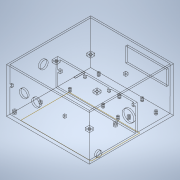
# Autodesk Inventor part: Base
Saved by Autodesk Inventor 2022.2 (Build 262287000, 287)
## iProperties
Created: 2022-01-15
Part Number: Base
Material: Generic
Document SubType Name: Modeling
Designer: siwat
Density: 1 g/cm^3
Appearance: Default
Author: siwat
Autodesk Inventor part; units mm, degrees
ref_plane "YZ Plane" through (0, 0, 0) normal (1, 0, 0) x (0, 1, 0)
ref_plane "XZ Plane" through (0, 0, 0) normal (0, 1, 0) x (-1, 0, 0)
ref_plane "XY Plane" through (0, 0, 0) normal (0, 0, 1) x (1, 0, 0)
ref_plane "Work Plane1" through (31.5112, 10.0003, 59.575) normal (-0.0015858, -0.9999987, 0.0000018) x (-0.0011293, 0, -0.9999994)
sketch "Sketch1" plane through (31.5112, 10.0003, 59.575) normal (-0.0015858, -0.9999987, 0.0000018) x (-0.0011293, 0, -0.9999994)
  line L0 (-4.5224, 4.5326) -> (134.4396, 4.5326)
  line L1 (134.4396, 4.5326) -> (134.4396, -131.8992)
  line L2 (134.4396, -131.8992) -> (-4.5224, -131.8992)
  line L3 (-4.5224, -131.8992) -> (-4.5224, 4.5326)
  line L4 (-7.5224, 7.5326) -> (137.4396, 7.5326)
  line L5 (137.4396, 7.5326) -> (137.4396, -134.8992)
  line L6 (137.4396, -134.8992) -> (-7.5224, -134.8992)
  line L7 (-7.5224, -134.8992) -> (-7.5224, 7.5326)
  point P0 (59.6106, -31.428)
  dimension "d0" = 138.9621
  dimension "d1" = 136.4319
  dimension "d2" = 74.8291
  dimension "d3" = 35.9607
  dimension "d4" = 3
  dimension "d5" = 3
  dimension "d6" = 3
  dimension "d7" = 3
  constraints: 16 end point, 4 parallel, 2 horizontal, 2 perpendicular
  measures "d0" distance between parallel lines of L1 L3
  measures "d1" distance between parallel lines of L0 L2
  measures "d2" distance from line of point (59.611, -31.428) L1
  measures "d3" distance from line of point (59.611, -31.428) L0
  measures "d4" distance between parallel lines of L0 L4
  measures "d5" distance between parallel lines of L3 L7
  measures "d6" distance between parallel lines of L5 L1
  measures "d7" distance between parallel lines of L6 L2
extrude "Extrusion1" add sketch "Sketch1" against normal blind 74.125
sketch "Sketch2" plane through (31.5112, 10.0003, 59.575) normal (-0.0015858, -0.9999987, 0.0000018) x (0.9999981, -0.0015858, -0.0011293)
  line L0 (-134.8992, -137.4396) -> (7.5326, -137.4396) projected
  line L1 (7.5326, 7.5224) -> (-134.8992, 7.5224) projected
  line L2 (7.5326, -137.4396) -> (-134.8992, -137.4396)
  line L3 (-134.8992, -137.4396) -> (-134.8992, 7.5224)
  line L4 (-134.8992, 7.5224) -> (7.5326, 7.5224)
  line L5 (7.5326, 7.5224) -> (7.5326, -137.4396)
  point P0 (-31.428, -59.6106)
  point P1 (-134.8992, -137.4396)
  point P2 (7.5326, 7.5224)
  constraints: 8 end point, 2 parallel, 1 horizontal, 1 perpendicular
extrude "Extrusion2" add sketch "Sketch2" along normal blind 3
sketch "Sketch3" plane through (31.5112, 10.0003, 59.575) normal (0.0015858, 0.9999987, -0.0000018) x (0.9999981, -0.0015858, -0.0011293)
  circle A0 centre (-112.8782, 129.2967) radius 1.9965
  circle A1 centre (-112.8782, 129.2967) radius 0.875
  circle A2 centre (-114.2274, 81.024) radius 1.9965
  circle A3 centre (-114.2274, 81.024) radius 0.875
  circle A4 centre (-62.1401, 86.0453) radius 1.9965
  circle A5 centre (-62.1401, 86.0453) radius 0.875
  circle A6 centre (-62.0938, 113.9832) radius 1.9965
  circle A7 centre (-62.0938, 113.9832) radius 0.875
  circle A8 centre (-37.9957, 129.2347) radius 1.9965
  circle A9 centre (-37.9957, 129.2347) radius 0.875
  circle A10 centre (-31.6312, 80.9446) radius 1.9965
  circle A11 centre (-31.6312, 80.9446) radius 0.875
  circle A12 centre (-6.6551, 121.5212) radius 2.3058
  circle A13 centre (-6.6551, 121.5212) radius 0.875
  circle A14 centre (-22.9352, 91.3493) radius 2.3058
  circle A15 centre (-22.9352, 91.3493) radius 0.875
  circle A16 centre (-129.08, 0.6108) radius 2.6932
  circle A17 centre (-129.08, 0.6108) radius 0.875
  circle A18 centre (-24.0772, 69.1234) radius 2.8442
  circle A19 centre (-24.0772, 69.1234) radius 0.875
  point P0 (-31.428, 59.6106)
  dimension "d12" = 1.75
  dimension "d13" = 1.75
  dimension "d14" = 1.75
  dimension "d15" = 1.75
  dimension "d16" = 1.75
  dimension "d17" = 1.75
  dimension "d18" = 1.75
  dimension "d19" = 1.75
  dimension "d28" = 1.75
  dimension "d29" = 1.75
  constraints: 20 centre point, 10 coincident
  measures "d12" diameter of A1
  measures "d13" diameter of A3
  measures "d14" diameter of A5
  measures "d15" diameter of A7
  measures "d16" diameter of A9
  measures "d17" diameter of A11
  measures "d18" diameter of A13
  measures "d19" diameter of A15
  measures "d28" diameter of A17
  measures "d29" diameter of A19
extrude "Extrusion3" add sketch "Sketch3" along normal blind 5
sketch "Sketch4" plane through (31.5112, 10.0003, 59.575) normal (0.0015858, 0.9999987, -0.0000018) x (0.9999981, -0.0015858, -0.0011293)
  line L0 (4.5326, 134.4396) -> (4.5326, -4.5224) projected
  line L1 (-131.8992, 134.4396) -> (-131.8992, -4.5224) projected
  line L2 (4.5326, 74.8611) -> (-131.8992, 74.8611)
  line L3 (-131.8992, 74.8611) -> (-131.8992, 77.8611)
  line L4 (-131.8992, 77.8611) -> (4.5326, 77.8611)
  line L5 (4.5326, 77.8611) -> (4.5326, 74.8611)
  point P0 (-31.428, 59.6106)
  point P1 (4.5326, 77.8611)
  point P2 (-131.8992, 74.8611)
  dimension "d22" = 3
  constraints: 8 end point, 2 parallel, 2 point on line, 1 horizontal, 1 perpendicular
  measures "d22" distance between parallel lines of L4 L2
extrude "Extrusion4" add sketch "Sketch4" along normal blind 45
sketch "Sketch5" plane through (35.9559, 9.9931, -18.2911) normal (-0.0011293, 0, -0.9999994) x (-0.9999981, 0.0015858, 0.0011293)
  circle A0 centre (12.779, 19.6609) radius 10
  point P0 (35.9607, -10.0501)
  dimension "d25" = 20
  constraints: 1 centre point
  measures "d25" diameter of A0
extrude "Extrusion5" cut sketch "Sketch5" against normal up to surface (3 mm away)
sketch "Sketch7" plane through (-100.5396, 10.2094, -74.7156) normal (0.9999981, -0.0015858, -0.0011293) x (-0.0011293, 0, -0.9999994)
  line L0 (0, 0) -> (0, 74.125) projected
  line L1 (0, 24.9377) -> (-4, 24.9377)
  line L2 (-4, 24.9377) -> (-4, 20.9377)
  line L3 (-4, 20.9377) -> (0, 20.9377)
  line L4 (0, 20.9377) -> (0, 24.9377)
  line L5 (-4, 24.9377) -> (-56.5786, 24.9377)
  line L6 (-56.5786, 45) -> (-56.5786, 0) projected
  line L7 (-4, 20.9377) -> (-56.5786, 20.9377)
  line L8 (-52.5786, 24.9377) -> (-52.5786, 20.9377)
  line L9 (-56.5786, 0) -> (-56.5786, 45) projected
  point P0 (-74.8291, -10.0501)
  point P1 (-56.5786, 90)
  dimension "d30" = 4
  dimension "d31" = 4
  dimension "d34" = 4
  constraints: 15 end point, 4 point on line, 3 horizontal, 2 parallel, 2 perpendicular
  measures "d30" distance of L3.end L2.end
  measures "d31" distance of L2.end L1.end
  measures "d34" distance from line of L6.start L8
extrude "Extrusion6" add sketch "Sketch7" along normal blind 4 contours L3 L2 L1 L0 | L7 L6 L5 L8
sketch "Sketch8" plane through (-100.4955, 35.1471, -70.7156) normal (0.0015858, 0.9999987, -0.0000018) x (0.9999981, -0.0015858, -0.0011293)
  line L0 (136.4319, 4) -> (136.4319, -134.9621) projected
  line L1 (136.4319, 4) -> (129.4319, 4)
  line L2 (129.4319, 4) -> (129.4319, -3)
  line L3 (129.4319, -3) -> (136.4319, -3)
  line L4 (136.4319, -3) -> (136.4319, 4)
  line L5 (136.4319, -52.5786) -> (132.4319, -52.5786)
  line L6 (132.4319, -52.5786) -> (132.4319, -48.5786)
  line L7 (132.4319, -48.5786) -> (136.4319, -48.5786)
  line L8 (136.4319, -48.5786) -> (136.4319, -52.5786)
  line L9 (136.4319, 4) -> (0, 4) projected
  line L10 (60.4128, 4) -> (64.4128, 4)
  line L11 (64.4128, 4) -> (64.4128, 0)
  line L12 (64.4128, 0) -> (60.4128, 0)
  line L13 (60.4128, 0) -> (60.4128, 4)
  line L14 (0, -52.5786) -> (136.4319, -52.5786) projected
  line L15 (60.4128, -52.5786) -> (67.4128, -52.5786)
  line L16 (67.4128, -52.5786) -> (67.4128, -45.5786)
  line L17 (67.4128, -45.5786) -> (60.4128, -45.5786)
  line L18 (60.4128, -45.5786) -> (60.4128, -52.5786)
  circle A0 centre (132.9319, 0.5) radius 1.25
  circle A1 centre (63.9128, -49.0786) radius 1.25
  point P0 (100.4712, -70.8291)
  point P1 (67.4128, -52.5786)
  point P2 (64.4128, 4)
  dimension "d35" = 7
  dimension "d36" = 7
  dimension "d37" = 4
  dimension "d38" = 4
  dimension "d39" = 4
  dimension "d40" = 4
  dimension "d41" = 7
  dimension "d42" = 7
  dimension "d45" = 2.5
  dimension "d46" = 3.5
  dimension "d47" = 3.5
  dimension "d48" = 2.5
  dimension "d49" = 3.5
  dimension "d50" = 3.5
  constraints: 32 end point, 8 parallel, 4 horizontal, 4 perpendicular, 3 point on line, 2 centre point
  measures "d35" distance of L3.end L2.end
  measures "d36" distance of L2.end L1.end
  measures "d37" distance of L6.end L7.end
  measures "d38" distance of L5.end L6.end
  measures "d39" distance of L11.end L12.end
  measures "d40" distance of L10.end L11.end
  measures "d41" distance of L17.end L16.end
  measures "d42" distance of L16.end L15.end
  measures "d45" diameter of A0
  measures "d46" distance from line of L9 A0.centre
  measures "d47" distance from line of L0 A0.centre
  measures "d48" diameter of A1
  measures "d49" distance from line of A1.centre L17
  measures "d50" distance from line of L16 A1.centre
extrude "Extrusion7" add sketch "Sketch8" against normal blind 4 contours L11 L12 L13 L9 | L18 L17 L16 L14
sketch "Sketch9" plane through (-100.4955, 35.1471, -70.7156) normal (0.0015858, 0.9999987, -0.0000018) x (0.9999981, -0.0015858, -0.0011293)
  line L0 (4, 4) -> (0, 4) projected
  line L1 (0, 4) -> (7, 4)
  line L2 (7, 4) -> (7, -3)
  line L3 (7, -3) -> (0, -3)
  line L4 (0, -3) -> (0, 4)
  point P0 (100.4712, -70.8291)
  point P1 (4, 4)
  dimension "d51" = 7
  dimension "d52" = 7
  constraints: 8 end point, 2 parallel, 1 horizontal, 1 perpendicular
  measures "d51" distance of L2.end L3.end
  measures "d52" distance of L1.end L2.end
extrude "Extrusion8" add sketch "Sketch9" against normal up to surface (4 mm away)
sketch "Sketch10" plane through (-100.4921, 35.1471, -67.7156) normal (0.0015858, 0.9999987, -0.0000018) x (0.9999981, -0.0015858, -0.0011293)
  circle A0 centre (3.5, 3.5) radius 1.25
  line L0 (0, -131.9621) -> (0, 7) projected
  line L1 (0, 0) -> (7, 0) projected
  point P0 (100.4712, -67.8291)
  point P1 (0, -49.5786)
  dimension "d55" = 2.5
  dimension "d56" = 3.5
  dimension "d57" = 3.5
  constraints: 1 centre point
  measures "d55" diameter of A0
  measures "d56" distance from line of L0 A0.centre
  measures "d57" distance from line of L1 A0.centre
extrude "Extrusion9" cut sketch "Sketch10" against normal up to surface (4 mm away)
sketch "Sketch11" plane through (31.5826, 55.0002, 59.5749) normal (0.0015858, 0.9999987, -0.0000018) x (0.9999981, -0.0015858, -0.0011293)
  line L0 (-131.8992, 74.8611) -> (-131.8992, 77.8611) projected
  line L1 (-131.8992, 74.8611) -> (-124.8992, 74.8611)
  line L2 (-124.8992, 74.8611) -> (-124.8992, 67.8611)
  line L3 (-124.8992, 67.8611) -> (-131.8992, 67.8611)
  line L4 (-131.8992, 67.8611) -> (-131.8992, 74.8611)
  line L5 (-131.8992, -4.5224) -> (4.5326, -4.5224) projected
  line L6 (4.5326, -4.5224) -> (-2.4674, -4.5224)
  line L7 (-2.4674, -4.5224) -> (-2.4674, 2.4776)
  line L8 (-2.4674, 2.4776) -> (4.5326, 2.4776)
  line L9 (4.5326, 2.4776) -> (4.5326, -4.5224)
  circle A0 centre (1.0326, -1.0224) radius 1.25
  circle A1 centre (-128.3992, 71.3611) radius 1.25
  line L10 (-131.8992, -4.5224) -> (-128.8992, -4.5224)
  line L11 (-128.8992, -4.5224) -> (-128.8992, -1.5224)
  line L12 (-128.8992, -1.5224) -> (-131.8992, -1.5224)
  line L13 (-131.8992, -1.5224) -> (-131.8992, -4.5224)
  line L14 (-131.8992, 74.8611) -> (4.5326, 74.8611) projected
  line L15 (4.5326, 74.8611) -> (1.5326, 74.8611)
  line L16 (1.5326, 74.8611) -> (1.5326, 71.8611)
  line L17 (1.5326, 71.8611) -> (4.5326, 71.8611)
  line L18 (4.5326, 71.8611) -> (4.5326, 74.8611)
  line L19 (-82.1632, -4.5224) -> (-79.1632, -4.5224)
  line L20 (-79.1632, -4.5224) -> (-79.1632, -1.5224)
  line L21 (-79.1632, -1.5224) -> (-82.1632, -1.5224)
  line L22 (-82.1632, -1.5224) -> (-82.1632, -4.5224)
  line L23 (4.5326, 74.8611) -> (-131.8992, 74.8611) projected
  line L24 (-82.1632, 74.8611) -> (-79.1632, 74.8611)
  line L25 (-79.1632, 74.8611) -> (-79.1632, 71.8611)
  line L26 (-79.1632, 71.8611) -> (-82.1632, 71.8611)
  line L27 (-82.1632, 71.8611) -> (-82.1632, 74.8611)
  line L28 (-40.7381, -4.5224) -> (-37.7381, -4.5224)
  line L29 (-37.7381, -4.5224) -> (-37.7381, -1.5224)
  line L30 (-37.7381, -1.5224) -> (-40.7381, -1.5224)
  line L31 (-40.7381, -1.5224) -> (-40.7381, -4.5224)
  line L32 (-40.7381, 74.8611) -> (-37.7381, 74.8611)
  line L33 (-37.7381, 74.8611) -> (-37.7381, 71.8611)
  line L34 (-37.7381, 71.8611) -> (-40.7381, 71.8611)
  line L35 (-40.7381, 71.8611) -> (-40.7381, 74.8611)
  point P0 (-31.428, 59.6106)
  point P1 (1.5326, 74.8611)
  point P2 (-2.4674, -4.5224)
  point P3 (-128.8992, -4.5224)
  point P4 (-37.7381, 74.8611)
  point P5 (-40.7381, 74.8611)
  point P6 (-79.1632, 74.8611)
  point P7 (-82.1632, 74.8611)
  point P8 (-79.1632, -4.5224)
  point P9 (-37.7381, -4.5224)
  dimension "d60" = 7
  dimension "d61" = 7
  dimension "d62" = 7
  dimension "d63" = 7
  dimension "d64" = 2.5
  dimension "d65" = 2.5
  dimension "d66" = 3
  dimension "d67" = 3
  dimension "d68" = 3
  dimension "d69" = 3
  dimension "d72" = 3
  dimension "d73" = 3
  dimension "d74" = 3
  dimension "d75" = 3
  dimension "d76" = 3
  dimension "d77" = 3
  dimension "d78" = 3
  dimension "d79" = 3
  constraints: 64 end point, 16 parallel, 8 horizontal, 8 perpendicular, 6 point on line, 2 centre point
  measures "d60" distance of L2.end L3.end
  measures "d61" distance of L1.end L2.end
  measures "d62" distance of L7.end L8.end
  measures "d63" distance of L6.end L7.end
  measures "d64" diameter of A0
  measures "d65" diameter of A1
  measures "d66" distance of L12.end L11.end
  measures "d67" distance of L11.end L10.end
  measures "d68" distance of L17.end L16.end
  measures "d69" distance of L16.end L15.end
  measures "d72" distance of L21.end L20.end
  measures "d73" distance of L20.end L19.end
  measures "d74" distance of L25.end L26.end
  measures "d75" distance of L24.end L25.end
  measures "d76" distance of L30.end L29.end
  measures "d77" distance of L29.end L28.end
  measures "d78" distance of L33.end L34.end
  measures "d79" distance of L32.end L33.end
extrude "Extrusion10" add sketch "Sketch11" against normal blind 4
sketch "Sketch12" plane through (39.1699, 84.1132, 67.0888) normal (0.9999981, -0.0015858, -0.0011293) x (-0.0011293, 0, -0.9999994)
  circle A0 centre (16.9004, -70.7033) radius 5
  point P0 (67.133, -84.1751)
  dimension "d80" = 10
  constraints: 1 centre point
  measures "d80" diameter of A0
extrude "Extrusion11" cut sketch "Sketch12" against normal up to surface (3 mm away)
sketch "Sketch13" plane through (-103.4254, 84.3391, -77.7123) normal (-0.9999981, 0.0015858, 0.0011293) x (0.0011293, 0, 0.9999994)
  line L0 (12.035, -76.8057) -> (29.035, -76.8057)
  line L1 (29.035, -76.8057) -> (29.035, -86.8057)
  line L2 (29.035, -86.8057) -> (12.035, -86.8057)
  line L3 (12.035, -86.8057) -> (12.035, -76.8057)
  point P0 (77.8291, -84.1751)
  dimension "d83" = 17
  dimension "d84" = 10
  constraints: 8 end point, 2 parallel, 1 horizontal, 1 perpendicular
  measures "d83" distance of L1.end L2.end
  measures "d84" distance of L0.end L1.end
extrude "Extrusion12" cut sketch "Sketch13" against normal up to surface (3 mm away)
sketch "Sketch14" plane through (-103.2617, 84.3391, 67.2497) normal (0.0011293, 0, 0.9999994) x (0.9999981, -0.0015858, -0.0011293)
  circle A0 centre (28.9462, -29.0559) radius 7
  circle A1 centre (50.0819, -32.0843) radius 7
  point P0 (103.4712, -84.1751)
  dimension "d87" = 14
  dimension "d88" = 14
  constraints: 2 centre point
  measures "d87" diameter of A0
  measures "d88" diameter of A1
extrude "Extrusion13" cut sketch "Sketch14" against normal up to surface (3 mm away)
sketch "Sketch15" plane through (-103.4254, 84.3391, -77.7123) normal (-0.9999981, 0.0015858, 0.0011293) x (0.0011293, 0, 0.9999994)
  circle A0 centre (83.1255, -29.8584) radius 7
  point P0 (77.8291, -84.1751)
  dimension "d91" = 14
  constraints: 1 centre point
  measures "d91" diameter of A0
extrude "Extrusion14" cut sketch "Sketch15" against normal up to surface (3 mm away)
sketch "Sketch16" plane through (39.0062, 84.1132, -77.8732) normal (-0.0011293, 0, -0.9999994) x (-0.9999981, 0.0015858, 0.0011293)
  line L0 (80.034, -10.8316) -> (8.5598, -10.8316)
  line L1 (8.5598, -10.8316) -> (8.5598, -37.8544)
  line L2 (8.5598, -37.8544) -> (80.034, -37.8544)
  line L3 (80.034, -37.8544) -> (80.034, -10.8316)
  point P0 (38.9607, -84.1751)
  constraints: 8 end point, 2 parallel, 1 horizontal, 1 perpendicular
extrude "Extrusion15" cut sketch "Sketch16" against normal up to surface (3 mm away)
equation "\"d5\" = d4"
equation "\"d6\" = d4"
equation "\"d7\" = d5"
equation "\"d46\" = 0.5 * d36"
equation "\"d47\" = 0.5 * d35"
equation "\"d49\" = 0.5 * d41"
equation "\"d50\" = 0.5 * d42"
body "Solid1"
